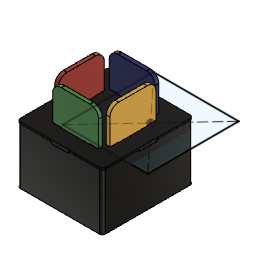
power supply box (Autodesk Fusion 360 design; units mm, degrees)
Autodesk Fusion 360 part; units mm, degrees
sketch "Sketch1" plane through (0, 0, 0) normal (0, 0, 1) x (1, 0, 0) in component "power supply"
  line L0 (-71.12, 76.2) -> (71.12, 76.2)
  line L1 (71.12, 76.2) -> (71.12, -76.2)
  line L2 (71.12, -76.2) -> (-71.12, -76.2)
  line L3 (-71.12, -76.2) -> (-71.12, 76.2)
  line L4 (-74.12, 79.2) -> (74.12, 79.2)
  line L5 (74.12, 79.2) -> (74.12, -79.2)
  line L6 (74.12, -79.2) -> (-74.12, -79.2)
  line L7 (-74.12, -79.2) -> (-74.12, 79.2)
  line L8 (-74.12, 79.2) -> (74.12, -79.2) construction
  line L9 (74.12, 79.2) -> (-74.12, -79.2) construction
  dimension "d4" = 142.24
  dimension "d5" = 152.4
  dimension "d25" = 148.24
  dimension "d26" = 158.4
  constraint horizontal L0
  constraint perpendicular L0 L1
  constraint parallel L0 L2
  constraint parallel L1 L3
  constraint horizontal L4
  constraint perpendicular L4 L5
  constraint parallel L4 L6
  constraint parallel L5 L7
  constraint coincident L8 origin
  constraint coincident L9 origin
  measures "d4" distance of L1.end L2.end
  measures "d5" distance of L0.end L1.end
  measures "d25" distance of L5.end L6.end
  measures "d26" distance of L4.end L5.end
combine "Combine1" [no effect] in component "power supply"
extrude "Extrude7" add sketch "Sketch1" against normal blind 3 contours L0 L1 L2 L3 | L4 L5 L6 L7 makes body 1 in component "power supply"
extrude "Extrude8" add sketch "Sketch1" along normal blind 91.694 bodies 1 in component "power supply"
sketch "Sketch4" plane through (0, 0, 91.694) normal (0, 0, 1) x (-1, 0, 0) in component "power supply"
  line L0 (-71.12, 76.2) -> (71.12, 76.2)
  line L1 (71.12, 76.2) -> (71.12, -76.2)
  line L2 (71.12, -76.2) -> (-71.12, -76.2)
  line L3 (-71.12, -76.2) -> (-71.12, 76.2)
  line L4 (74.12, 79.2) -> (-74.12, 79.2)
  line L5 (-74.12, 79.2) -> (-74.12, -79.2)
  line L6 (-74.12, -79.2) -> (74.12, -79.2)
  line L7 (74.12, -79.2) -> (74.12, 79.2)
  line L8 (15, -76.2) -> (-15, -76.2)
  line L9 (-15, -76.2) -> (-15, -82.2)
  line L10 (-15, -82.2) -> (15, -82.2)
  line L11 (15, -82.2) -> (15, -76.2)
  line L12 (15, -76.2) -> (-15, -82.2) construction
  line L13 (-15, -76.2) -> (15, -82.2) construction
  line L14 (71.12, -15) -> (77.12, -15)
  line L15 (77.12, -15) -> (77.12, 15)
  line L16 (77.12, 15) -> (71.12, 15)
  line L17 (71.12, 15) -> (71.12, -15)
  line L18 (71.12, -15) -> (77.12, 15) construction
  line L19 (77.12, -15) -> (71.12, 15) construction
  line L20 (-71.12, -15) -> (-77.12, -15)
  line L21 (-77.12, -15) -> (-77.12, 15)
  line L22 (-77.12, 15) -> (-71.12, 15)
  line L23 (-71.12, 15) -> (-71.12, -15)
  line L24 (-71.12, -15) -> (-77.12, 15) construction
  line L25 (-77.12, -15) -> (-71.12, 15) construction
  line L26 (15, 76.2) -> (-15, 76.2)
  line L27 (-15, 76.2) -> (-15, 82.2)
  line L28 (-15, 82.2) -> (15, 82.2)
  line L29 (15, 82.2) -> (15, 76.2)
  line L30 (15, 76.2) -> (-15, 82.2) construction
  line L31 (-15, 76.2) -> (15, 82.2) construction
  point P0 (0, -79.2)
  point P1 (74.12, 0)
  point P2 (-74.12, 0)
  point P3 (0, 79.2)
  dimension "d31" = 30
  dimension "d32" = 6
  dimension "d33" = 30
  dimension "d34" = 30
  dimension "d35" = 30
  constraint horizontal L8
  constraint perpendicular L8 L9
  constraint parallel L8 L10
  constraint parallel L9 L11
  constraint coincident L12 P0
  constraint coincident L13 P0
  constraint midpoint L6 P0
  constraint horizontal L14
  constraint perpendicular L14 L15
  constraint parallel L14 L16
  constraint parallel L15 L17
  constraint coincident L18 P1
  constraint coincident L19 P1
  constraint midpoint L7 P1
  constraint horizontal L20
  constraint perpendicular L20 L21
  constraint parallel L20 L22
  constraint parallel L21 L23
  constraint coincident L24 P2
  constraint coincident L25 P2
  constraint midpoint L5 P2
  constraint horizontal L26
  constraint perpendicular L26 L27
  constraint parallel L26 L28
  constraint parallel L27 L29
  constraint coincident L30 P3
  constraint coincident L31 P3
  constraint midpoint L4 P3
  measures "d31" distance of L9.end L10.end
  measures "d32" distance of L8.end L9.end
  measures "d33" distance of L14.end L15.end
  measures "d34" distance of L20.end L21.end
  measures "d35" distance of L27.end L28.end
extrude "Extrude11" add sketch "Sketch4" along normal blind 3 separate body contours L0 L4 L26 L27 L29 | L3 L5 L20 L22 L23 | L1 L7 L14 L16 L17 | L2 L6 L8 L9 L11 makes body 2 at (5, -78.2, 91.694) makes body 3 at (5, 78.2, 91.694) makes body 4 at (-74.12, 5, 93.694) makes body 5 at (73.12, -5, 91.694) in component "power supply"
extrude "Extrude9" add sketch "Sketch4" along normal blind 3 contours L0 L3 L4 L5 L22 L27 | L0 L1 L4 L7 L16 L29 | L2 L3 L5 L6 L9 L20 | L1 L2 L6 L7 L11 L14 bodies 1 in component "power supply"
fillet "Fillet1" radius 5 4 edges at (-74.12, -79.2, 45.847) (74.12, -79.2, 45.847) (74.12, 79.2, 45.847) (-74.12, 79.2, 45.847) on bodies 1 in component "power supply"
sketch "Sketch1 (2)" plane through (0, 0, 94.694) normal (0, 0, 1) x (-1, 0, 0)
  arc A0 (-69.12, 79.2) -> (-74.12, 74.2) centre (-69.12, 74.2) ccw
  line L0 (-74.12, 74.2) -> (-74.12, 15)
  line L1 (-74.12, 15) -> (-71.12, 15)
  line L2 (-71.12, 15) -> (-71.12, 76.2)
  line L3 (-71.12, 76.2) -> (-15, 76.2)
  line L4 (-15, 76.2) -> (-15, 79.2)
  line L5 (-15, 79.2) -> (-69.12, 79.2)
  line L6 (74.12, 79.2) -> (-74.12, 79.2)
  line L7 (-74.12, 79.2) -> (-74.12, -79.2)
  line L8 (-74.12, -79.2) -> (74.12, -79.2)
  line L9 (74.12, -79.2) -> (74.12, 79.2)
  line L10 (74.12, 79.2) -> (-74.12, -79.2) construction
  line L11 (-74.12, 79.2) -> (74.12, -79.2) construction
  dimension "d42" = 148.24
  dimension "d43" = 158.4
  constraint horizontal L6
  constraint perpendicular L6 L7
  constraint parallel L6 L8
  constraint parallel L7 L9
  constraint coincident L10 origin
  constraint coincident L11 origin
  measures "d42" distance of L7.end L8.end
  measures "d43" distance of L6.end L7.end
extrude "Extrude1" add sketch "Sketch1 (2)" along normal blind 3 separate body contours A0 L0 L1 L2 L3 L4 L5 L6 L7 | L1 L2 L3 L4 L6 L7 L8 L9 makes body 6
fillet "Fillet1'" radius 5 1 edges at (-74.12, -79.2, 96.194) on bodies 6
fillet "Fillet2" radius 5 1 edges at (74.12, 79.2, 96.194) on bodies 6
fillet "Fillet3" radius 5 1 edges at (-74.12, 79.2, 96.194) on bodies 6
combine "Combine2" operation add target body 2 tool bodies 4 3 5 6 in component "power supply"
move_face "OffsetFaces1" offset -0.5 2 faces at (-15, 78.2, 92.694) (-72.12, 15, 92.694) on bodies 2 in component "power supply"
move_face "OffsetFaces2" offset -0.5 2 faces at (-15, -78.2, 92.694) (-73.12, -15, 92.694) on bodies 2 in component "power supply"
move_face "OffsetFaces3" offset -0.5 2 faces at (15, -77.2, 92.694) (73.12, -15, 92.694) on bodies 2 in component "power supply"
move_face "OffsetFaces4" offset -0.5 2 faces at (72.12, 15, 92.694) (15, 77.2, 92.694) on bodies 2 in component "power supply"
sketch "Sketch5" plane through (0, 0, 97.694) normal (0, 0, 1) x (-1, 0, 0) in component "power supply"
  arc A0 (69.12, -79.2) -> (74.12, -74.2) centre (69.12, -74.2) ccw
  line L0 (74.12, -74.2) -> (74.12, 74.2)
  arc A1 (74.12, 74.2) -> (69.12, 79.2) centre (69.12, 74.2) ccw
  line L1 (69.12, 79.2) -> (-69.12, 79.2)
  arc A2 (-69.12, 79.2) -> (-74.12, 74.2) centre (-69.12, 74.2) ccw
  line L2 (-74.12, 74.2) -> (-74.12, -74.2)
  arc A3 (-74.12, -74.2) -> (-69.12, -79.2) centre (-69.12, -74.2) ccw
  line L3 (-69.12, -79.2) -> (69.12, -79.2)
  line L4 (25, -46.825) -> (-25, -46.825)
  line L5 (-25, -46.825) -> (-25, -53.175)
  line L6 (-25, -53.175) -> (25, -53.175)
  line L7 (25, -53.175) -> (25, -46.825)
  line L8 (25, -46.825) -> (-25, -53.175) construction
  line L9 (-25, -46.825) -> (25, -53.175) construction
  line L10 (-25, 53.175) -> (25, 46.825) construction
  line L11 (25, 53.175) -> (-25, 46.825) construction
  line L12 (25, 53.175) -> (-25, 53.175)
  line L13 (-25, 53.175) -> (-25, 46.825)
  line L14 (25, 46.825) -> (25, 53.175)
  line L15 (-25, 46.825) -> (25, 46.825)
  line L16 (48.175, -25) -> (41.825, 25) construction
  line L17 (48.175, 25) -> (41.825, 25)
  line L18 (48.175, 25) -> (41.825, -25) construction
  line L19 (41.825, -25) -> (48.175, -25)
  line L20 (41.825, 25) -> (41.825, -25)
  line L21 (48.175, -25) -> (48.175, 25)
  line L22 (-48.175, 25) -> (-48.175, -25)
  line L23 (-41.825, 25) -> (-48.175, -25) construction
  line L24 (-41.825, -25) -> (-41.825, 25)
  line L25 (-48.175, -25) -> (-41.825, -25)
  line L26 (-41.825, 25) -> (-48.175, 25)
  line L27 (-41.825, -25) -> (-48.175, 25) construction
  point P0 (0, -50)
  point P1 (0, 50)
  point P2 (45, 0)
  point P3 (-45, 0)
  dimension "d69" = 50
  dimension "d70" = 6.35
  dimension "d71" = 50
  dimension "d72" = 6.35
  dimension "d73" = 50
  dimension "d74" = 6.35
  dimension "d75" = 50
  dimension "d76" = 6.35
  constraint horizontal L4
  constraint perpendicular L4 L5
  constraint parallel L4 L6
  constraint parallel L5 L7
  constraint coincident L8 P0
  constraint coincident L9 P0
  constraint horizontal L12
  constraint perpendicular L12 L13
  constraint parallel L12 L15
  constraint parallel L13 L14
  constraint coincident P1 L11
  constraint coincident P1 L10
  constraint perpendicular L17 L21
  constraint parallel L20 L21
  constraint parallel L17 L19
  constraint coincident P2 L16
  constraint coincident P2 L18
  constraint perpendicular L24 L26
  constraint parallel L22 L24
  constraint parallel L25 L26
  constraint coincident P3 L27
  constraint coincident P3 L23
  measures "d69" distance of L5.end L6.end
  measures "d70" distance of L4.end L5.end
  measures "d71" distance of L11.end L10.end
  measures "d72" distance of L10.start L11.end
  measures "d73" distance of L16.end L18.end
  measures "d74" distance of L17.start L16.end
  measures "d75" distance of L22.end L22.start
  measures "d76" distance of L23.start L22.start
extrude "Extrude13" cut sketch "Sketch5" against normal blind 20 contours L4 L5 L6 L7 | L12 L13 L14 L15 | L17 L19 L20 L21 | L22 L24 L25 L26 bodies 2 in component "power supply"
sketch "Sketch1 (3)" plane through (0, 0, 112.2907) normal (0, 0, 1) x (-1, 0, 0) in component "acrylic"
  line L0 (70.9111, 75.088) -> (77.2611, 75.088)
  line L1 (77.2611, 75.088) -> (77.2611, 25.088)
  line L2 (77.2611, 25.088) -> (70.9111, 25.088)
  line L3 (70.9111, 25.088) -> (70.9111, 75.088)
  line L4 (-19.0889, 25.088) -> (-19.0889, 75.088)
  line L5 (-19.0889, 75.088) -> (-12.7389, 75.088)
  line L6 (-12.7389, 75.088) -> (-12.7389, 25.088)
  line L7 (-12.7389, 25.088) -> (-19.0889, 25.088)
  line L8 (4.0861, 3.263) -> (54.0861, 3.263)
  line L9 (54.0861, 3.263) -> (54.0861, -3.087)
  line L10 (54.0861, -3.087) -> (4.0861, -3.087)
  line L11 (4.0861, -3.087) -> (4.0861, 3.263)
  line L12 (54.0861, 103.263) -> (54.0861, 96.913)
  line L13 (54.0861, 96.913) -> (4.0861, 96.913)
  line L14 (4.0861, 96.913) -> (4.0861, 103.263)
  line L15 (4.0861, 103.263) -> (54.0861, 103.263)
  arc A0 (98.2061, -29.112) -> (103.2061, -24.112) centre (98.2061, -24.112) ccw
  line L16 (103.2061, -24.112) -> (103.2061, 124.288)
  arc A1 (103.2061, 124.288) -> (98.2061, 129.288) centre (98.2061, 124.288) ccw
  line L17 (98.2061, 129.288) -> (-40.0339, 129.288)
  arc A2 (-40.0339, 129.288) -> (-45.0339, 124.288) centre (-40.0339, 124.288) ccw
  line L18 (-45.0339, 124.288) -> (-45.0339, -24.112)
  arc A3 (-45.0339, -24.112) -> (-40.0339, -29.112) centre (-40.0339, -24.112) ccw
  line L19 (-40.0339, -29.112) -> (98.2061, -29.112)
  line L20 (35, -200) -> (-15, -200)
  line L21 (-30, -185) -> (-30, -140)
  line L22 (50, -140) -> (50, -185)
  line L23 (-15, -140) -> (-15, -135)
  line L24 (-15, -135) -> (35, -135)
  line L25 (35, -135) -> (35, -140)
  line L26 (-30, -140) -> (-15, -140)
  line L27 (35, -140) -> (50, -140)
  arc A4 (35, -200) -> (50, -185) centre (35, -185) ccw
  arc A5 (-30, -185) -> (-15, -200) centre (-15, -185) ccw
  point P0 (50, -200)
  point P1 (-30, -200)
  dimension "d80" = 80
  dimension "d81" = 60
  dimension "d82" = 50
  dimension "d83" = 5
  dimension "d84" = 15
  dimension "d85" = 15
  constraint horizontal L20
  constraint vertical L21
  constraint horizontal L26
  constraint vertical L22
  constraint vertical L23
  constraint horizontal L24
  constraint vertical L25
  constraint coincident L25.end L26
  constraint collinear L26 L27
  constraint coincident P0 L20
  constraint coincident P0 L22
  constraint tangent L20 A4
  constraint tangent L22 A4
  constraint coincident P1 L20
  constraint coincident P1 L21
  constraint tangent L20 A5
  constraint tangent L21 A5
  measures "d80" distance of P0 P1
  measures "d81" distance of P0 L22.start
  measures "d82" distance of L25.end L23.start
  measures "d83" distance of L25.end L24.end
  measures "d84" radius of A4
  measures "d85" radius of A5
extrude "Extrude1'" add sketch "Sketch1 (3)" along normal blind 6.35 separate body contours L20 L21 L22 L23 L24 L25 L26 L27 A4 A5 makes body 7 in component "acrylic"
move_body "Move3" bodies 2 to x (1, 0, 0) y (0, 1, 0) z (0, 0, 1) at (-160, 0, 0) in component "power supply"
sketch "Sketch2" plane through (0, 0, 109.2907) normal (0, 0, -1) x (1, 0, 0)
  line L0 (-237.2611, 75.088) -> (-230.9111, 75.088)
  line L1 (-230.9111, 75.088) -> (-230.9111, 25.088)
  line L2 (-230.9111, 25.088) -> (-237.2611, 25.088)
  line L3 (-237.2611, 25.088) -> (-237.2611, 75.088)
  line L4 (-140.9111, 75.088) -> (-140.9111, 25.088)
  line L5 (-140.9111, 25.088) -> (-147.2611, 25.088)
  line L6 (-147.2611, 25.088) -> (-147.2611, 75.088)
  line L7 (-147.2611, 75.088) -> (-140.9111, 75.088)
  line L8 (-214.0861, 3.263) -> (-164.0861, 3.263)
  line L9 (-164.0861, 3.263) -> (-164.0861, -3.087)
  line L10 (-164.0861, -3.087) -> (-214.0861, -3.087)
  line L11 (-214.0861, -3.087) -> (-214.0861, 3.263)
  line L12 (-203.5861, -29.112) -> (-203.5861, -26.112)
  line L13 (-203.5861, -26.112) -> (-174.5861, -26.112)
  line L14 (-174.5861, -26.112) -> (-174.5861, -29.112)
  line L15 (-174.5861, -29.112) -> (-119.9661, -29.112)
  arc A0 (-119.9661, -29.112) -> (-114.9661, -24.112) centre (-119.9661, -24.112) ccw
  line L16 (-114.9661, -24.112) -> (-114.9661, 35.588)
  line L17 (-114.9661, 35.588) -> (-117.9661, 35.588)
  line L18 (-117.9661, 35.588) -> (-117.9661, 64.588)
  line L19 (-117.9661, 64.588) -> (-114.9661, 64.588)
  line L20 (-114.9661, 64.588) -> (-114.9661, 124.288)
  arc A1 (-114.9661, 124.288) -> (-119.9661, 129.288) centre (-119.9661, 124.288) ccw
  line L21 (-119.9661, 129.288) -> (-174.5861, 129.288)
  line L22 (-174.5861, 129.288) -> (-174.5861, 126.288)
  line L23 (-174.5861, 126.288) -> (-203.5861, 126.288)
  line L24 (-203.5861, 126.288) -> (-203.5861, 129.288)
  line L25 (-203.5861, 129.288) -> (-258.2061, 129.288)
  arc A2 (-258.2061, 129.288) -> (-263.2061, 124.288) centre (-258.2061, 124.288) ccw
  line L26 (-263.2061, 124.288) -> (-263.2061, 64.588)
  line L27 (-263.2061, 64.588) -> (-260.2061, 64.588)
  line L28 (-260.2061, 64.588) -> (-260.2061, 35.588)
  line L29 (-260.2061, 35.588) -> (-263.2061, 35.588)
  line L30 (-263.2061, 35.588) -> (-263.2061, -24.112)
  arc A3 (-263.2061, -24.112) -> (-258.2061, -29.112) centre (-258.2061, -24.112) ccw
  line L31 (-258.2061, -29.112) -> (-203.5861, -29.112)
  line L32 (-213.9087, 107.7569) -> (-164.2635, 107.7569)
  line L33 (-164.2635, 107.7569) -> (-164.2635, 91.7569)
  line L34 (-164.2635, 91.7569) -> (-213.9087, 91.7569)
  line L35 (-213.9087, 91.7569) -> (-213.9087, 107.7569)
  line L36 (-213.9087, 107.7569) -> (-164.2635, 91.7569) construction
  line L37 (-164.2635, 107.7569) -> (-213.9087, 91.7569) construction
  line L38 (-164.2635, 107.7569) -> (-213.9087, 107.7569)
  line L39 (-213.9087, 107.7569) -> (-213.9087, 104.7569)
  line L40 (-213.9087, 104.7569) -> (-164.2635, 104.7569)
  line L41 (-164.2635, 104.7569) -> (-164.2635, 107.7569)
  line L42 (-213.9087, 91.7569) -> (-164.2635, 91.7569)
  line L43 (-164.2635, 91.7569) -> (-164.2635, 94.7569)
  line L44 (-164.2635, 94.7569) -> (-213.9087, 94.7569)
  line L45 (-213.9087, 94.7569) -> (-213.9087, 91.7569)
  line L46 (-136.2375, 25.1852) -> (-152.2375, 74.8304) construction
  line L47 (-152.2375, 74.8304) -> (-136.2375, 74.8304)
  line L48 (-152.2375, 74.8304) -> (-152.2375, 25.1852)
  line L49 (-149.2375, 74.8304) -> (-152.2375, 74.8304)
  line L50 (-139.2375, 74.8304) -> (-139.2375, 25.1852)
  line L51 (-136.2375, 25.1852) -> (-152.2375, 25.1852)
  line L52 (-136.2375, 74.8304) -> (-136.2375, 25.1852)
  line L53 (-136.2375, 74.8304) -> (-139.2375, 74.8304)
  line L54 (-149.2375, 25.1852) -> (-149.2375, 74.8304)
  line L55 (-139.2375, 25.1852) -> (-136.2375, 25.1852)
  line L56 (-152.2375, 25.1852) -> (-149.2375, 25.1852)
  line L57 (-136.2375, 25.1852) -> (-136.2375, 74.8304)
  line L58 (-136.2375, 74.8304) -> (-152.2375, 25.1852) construction
  line L59 (-152.2375, 25.1852) -> (-152.2375, 74.8304)
  line L60 (-226.2375, 25.1852) -> (-226.2375, 74.8304)
  line L61 (-229.2375, 74.8304) -> (-229.2375, 25.1852)
  line L62 (-229.2375, 25.1852) -> (-226.2375, 25.1852)
  line L63 (-226.2375, 74.8304) -> (-229.2375, 74.8304)
  line L64 (-242.2375, 74.8304) -> (-226.2375, 74.8304)
  line L65 (-239.2375, 25.1852) -> (-239.2375, 74.8304)
  line L66 (-242.2375, 25.1852) -> (-242.2375, 74.8304)
  line L67 (-226.2375, 25.1852) -> (-242.2375, 74.8304) construction
  line L68 (-226.2375, 74.8304) -> (-242.2375, 25.1852) construction
  line L69 (-226.2375, 25.1852) -> (-242.2375, 25.1852)
  line L70 (-242.2375, 74.8304) -> (-242.2375, 25.1852)
  line L71 (-239.2375, 74.8304) -> (-242.2375, 74.8304)
  line L72 (-226.2375, 74.8304) -> (-226.2375, 25.1852)
  line L73 (-242.2375, 25.1852) -> (-239.2375, 25.1852)
  line L74 (-164.2635, 4.7569) -> (-164.2635, 7.7569)
  line L75 (-213.9087, 7.7569) -> (-213.9087, 4.7569)
  line L76 (-213.9087, -8.2431) -> (-213.9087, 7.7569)
  line L77 (-213.9087, -8.2431) -> (-164.2635, -8.2431)
  line L78 (-164.2635, 7.7569) -> (-164.2635, -8.2431)
  line L79 (-213.9087, 4.7569) -> (-164.2635, 4.7569)
  line L80 (-164.2635, -5.2431) -> (-213.9087, -5.2431)
  line L81 (-213.9087, 7.7569) -> (-164.2635, 7.7569)
  line L82 (-164.2635, 7.7569) -> (-213.9087, -8.2431) construction
  line L83 (-213.9087, -5.2431) -> (-213.9087, -8.2431)
  line L84 (-164.2635, -8.2431) -> (-164.2635, -5.2431)
  line L85 (-164.2635, -8.2431) -> (-213.9087, -8.2431)
  line L86 (-164.2635, 7.7569) -> (-213.9087, 7.7569)
  line L87 (-213.9087, 7.7569) -> (-164.2635, -8.2431) construction
  point P0 (-189.0861, 99.7569)
  point P1 (-144.2375, 50.0078)
  point P2 (-234.2375, 50.0078)
  point P3 (-189.0861, -0.2431)
  dimension "d90" = 16
  dimension "d91" = 3
  dimension "d92" = 3
  dimension "d93" = 16
  dimension "d94" = 3
  dimension "d95" = 3
  dimension "d96" = 16
  dimension "d97" = 3
  dimension "d98" = 3
  dimension "d99" = 16
  dimension "d100" = 3
  dimension "d101" = 3
  constraint horizontal L32
  constraint perpendicular L32 L33
  constraint parallel L32 L34
  constraint parallel L33 L35
  constraint coincident L36 P0
  constraint coincident L37 P0
  constraint horizontal L38
  constraint vertical L39
  constraint horizontal L40
  constraint vertical L41
  constraint horizontal L42
  constraint vertical L43
  constraint horizontal L44
  constraint vertical L45
  constraint perpendicular L51 L52
  constraint parallel L52 L59
  constraint parallel L47 L51
  constraint coincident P1 L58
  constraint coincident P1 L46
  constraint perpendicular L69 L72
  constraint parallel L66 L72
  constraint parallel L64 L69
  constraint coincident P2 L68
  constraint coincident P2 L67
  constraint horizontal L81
  constraint perpendicular L78 L81
  constraint parallel L81 L85
  constraint parallel L76 L78
  constraint coincident P3 L87
  constraint coincident P3 L82
  constraint horizontal L86
  constraint vertical L75
  constraint horizontal L79
  constraint vertical L74
  constraint horizontal L77
  constraint vertical L84
  constraint horizontal L80
  constraint vertical L83
  measures "d90" distance of L32.end L33.end
  measures "d91" distance of L32.end L40.end
  measures "d92" distance of L34.end L44.end
  measures "d93" distance of L48.end L46.start
  measures "d94" distance of L50.end L46.start
  measures "d95" distance of L46.end L49.start
  measures "d96" distance of L66.start L60.start
  measures "d97" distance of L60.start L61.end
  measures "d98" distance of L65.end L64.start
  measures "d99" distance of L77.end L74.end
  measures "d100" distance of L74.start L74.end
  measures "d101" distance of L76.start L80.end
extrude "Extrude14" add sketch "Sketch2" along normal blind 5 contours L64 L65 L66 L69 L70 L71 L73 | L60 L61 L62 L63 L64 L69 L72 | L47 L50 L51 L52 L53 L55 L57 | L47 L48 L49 L51 L54 L56 L59 | L74 L75 L76 L78 L79 L81 L86 | L76 L77 L78 L80 L83 L84 L85 | L32 L33 L35 L38 L39 L40 L41 | L33 L34 L35 L42 L43 L44 L45 sketch seen with x (1, 0, 0) y (0, 1, 0) z (0, 0, 1) at (29.0861, 50.088, -14.5967) bodies 2 in component "power supply"
move_body "Move4" bodies 2 to x (1, 0, 0) y (0, 1, 0) z (0, 0, 1) at (150, 0, 0) in component "power supply"
move_body "Move5" bodies 2 to x (1, 0, 0) y (0, 1, 0) z (0, 0, 1) at (10, 0, 0) in component "power supply"
component "power supply" placed x (1, 0, 0) y (0, 1, 0) z (0, 0, 1) at (-29.0861, -50.088, 14.5967)
component "acrylic" placed x (1, 0, 0) y (0, 0, 1) z (0, -1, 0) at (-18.1407, 15.8701, -27.1597)
component "acrylic" placed x (1, 0, 0) y (0, 0, 1) z (0, -1, 0) at (-19, 115.3308, -26.8338)
component "acrylic" placed x (0, 1, 0) y (0, 0, 1) z (1, 0, 0) at (-189.4657, -40.1349, -26.8338)
component "acrylic" placed x (0, 1, 0) y (0, 0, 1) z (1, 0, 0) at (-99.4657, -40.1349, -26.8338)
equation "PSLength = 6 in"
equation "PSWidth = 5.6 in"
equation "PSHeight = 3.61 in"
equation "d4 = PSWidth"
equation "d5 = PSLength"
equation "casethick = 3 mm"
equation "d25 = PSWidth + 2 * casethick"
equation "d26 = PSLength + 2 * casethick"
equation "d27 = -casethick"
equation "d29 = PSHeight"
equation "d36 = casethick"
equation "d42 = PSWidth + 2 * casethick"
equation "d43 = PSLength + 2 * casethick"
equation "d44 = casethick"
equation "extra = 0.5 mm"
equation "d52 = -extra"
equation "d53 = -extra"
equation "d54 = -extra"
equation "d55 = -extra"
equation "acrylic = ( 1 / 4 ) * 1 in"
equation "acryliclength = 80 mm"
equation "acrylicgap = 50 mm"
equation "d69 = acrylicgap"
equation "d70 = acrylic"
equation "d71 = acrylicgap"
equation "d72 = acrylic"
equation "d73 = acrylicgap"
equation "d74 = acrylic"
equation "d75 = acrylicgap"
equation "d76 = acrylic"
equation "acrylicheight = 60 mm"
equation "d80 = acryliclength"
equation "d81 = acrylicheight"
equation "d82 = acrylicgap"
equation "d86 = acrylic"
equation "neopixelheight = 3 mm"
named bodies: "case", "lid"
